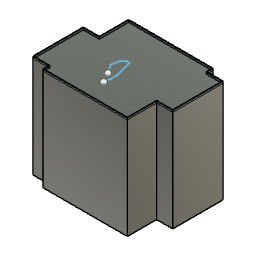
RSM_3d_model v1 (Autodesk Fusion 360 design; units mm, degrees)
Autodesk Fusion 360 part; units mm, degrees
sketch "Sketch1" plane through (0, 0, 0) normal (0, 0, 1) x (1, 0, 0)
sketch "Sketch2" plane through (0, 0, 0) normal (0, 0, 1) x (1, 0, 0)
  line L0 (106.508, 35.5843) -> (319.36, 35.5843)
  line L1 (106.508, 35.5843) -> (106.508, 50.8243)
  line L2 (106.508, 50.8243) -> (65.868, 50.8243)
  line L3 (65.868, 50.8243) -> (65.868, 177.8243)
  line L4 (65.868, 177.8243) -> (106.508, 177.8243)
  line L5 (106.508, 177.8243) -> (106.508, 251.4843)
  line L6 (106.508, 251.4843) -> (319.36, 251.4843)
  line L7 (319.36, 251.4843) -> (319.36, 236.2443)
  line L8 (319.36, 236.2443) -> (360, 236.2443)
  line L9 (360, 236.2443) -> (360, 109.2443)
  line L10 (360, 109.2443) -> (319.36, 109.2443)
  line L11 (319.36, 109.2443) -> (319.36, 35.5843)
  dimension "d2" = 212.852
  dimension "d3" = 15.24
  dimension "d4" = 40.64
  dimension "d5" = 127
  dimension "d6" = 40.64
  dimension "d7" = 73.66
  dimension "d8" = 212.852
  dimension "d9" = 15.24
  dimension "d10" = 40.64
  dimension "d11" = 73.66
  constraint horizontal L0
  constraint perpendicular L0 L1
  constraint perpendicular L1 L2
  constraint perpendicular L2 L3
  constraint perpendicular L3 L4
  constraint perpendicular L4 L5
  constraint perpendicular L5 L6
  constraint perpendicular L6 L7
  constraint perpendicular L7 L8
  constraint perpendicular L8 L9
  constraint perpendicular L9 L10
  constraint perpendicular L0 L11
  measures "d2" distance of L0.start L0.end
  measures "d3" distance of L0.start L1.end
  measures "d4" distance of L1.end L2.end
  measures "d5" distance of L2.end L3.end
  measures "d6" distance of L3.end L4.end
  measures "d7" distance of L4.end L5.end
  measures "d8" distance of L5.end L6.end
  measures "d9" distance of L6.end L7.end
  measures "d10" distance of L7.end L8.end
  measures "d11" distance of L0.end L10.end
extrude "Extrude1" add sketch "Sketch2" along normal blind 254
sketch "Sketch3" plane through (0, 0, 254) normal (0, 0, 1) x (-1, 0, 0)
  line L0 (-106.508, -35.5843) -> (-319.36, -35.5843)
  line L1 (-319.36, -35.5843) -> (-319.36, -109.2443)
  line L2 (-319.36, -109.2443) -> (-360, -109.2443)
  line L3 (-360, -109.2443) -> (-360, -236.2443)
  line L4 (-360, -236.2443) -> (-319.36, -236.2443)
  line L5 (-319.36, -236.2443) -> (-319.36, -251.4843)
  line L6 (-319.36, -251.4843) -> (-106.508, -251.4843)
  line L7 (-106.508, -251.4843) -> (-106.508, -177.8243)
  line L8 (-106.508, -177.8243) -> (-65.868, -177.8243)
  line L9 (-65.868, -177.8243) -> (-65.868, -50.8243)
  line L10 (-65.868, -50.8243) -> (-106.508, -50.8243)
  line L11 (-106.508, -50.8243) -> (-106.508, -35.5843)
  line L12 (-65.868, -177.8243) -> (-66.868, -177.8243)
  line L13 (-66.868, -177.8243) -> (-66.868, -50.8243)
  line L14 (-66.868, -50.8243) -> (-65.868, -50.8243)
  line L15 (-65.868, -50.8243) -> (-65.868, -177.8243)
  line L16 (-65.868, -177.8243) -> (-107.508, -177.8243)
  line L17 (-107.508, -177.8243) -> (-107.508, -176.8243)
  line L18 (-107.508, -176.8243) -> (-65.868, -176.8243)
  line L19 (-65.868, -176.8243) -> (-65.868, -177.8243)
  line L20 (-65.868, -50.8243) -> (-107.508, -50.8243)
  line L21 (-107.508, -50.8243) -> (-107.508, -51.8243)
  line L22 (-107.508, -51.8243) -> (-65.868, -51.8243)
  line L23 (-65.868, -51.8243) -> (-65.868, -50.8243)
  line L24 (-107.508, -51.8243) -> (-106.508, -51.8243)
  line L25 (-106.508, -51.8243) -> (-106.508, -35.5843)
  line L26 (-106.508, -35.5843) -> (-107.508, -35.5843)
  line L27 (-107.508, -35.5843) -> (-107.508, -51.8243)
  line L28 (-106.508, -35.5843) -> (-319.36, -35.5843)
  line L29 (-319.36, -35.5843) -> (-319.36, -36.5843)
  line L30 (-319.36, -36.5843) -> (-106.508, -36.5843)
  line L31 (-106.508, -36.5843) -> (-106.508, -35.5843)
  line L32 (-319.36, -35.5843) -> (-318.36, -35.5843)
  line L33 (-318.36, -35.5843) -> (-318.36, -110.2443)
  line L34 (-318.36, -110.2443) -> (-319.36, -110.2443)
  line L35 (-319.36, -110.2443) -> (-319.36, -35.5843)
  line L36 (-318.36, -110.2443) -> (-360, -110.2443)
  line L37 (-360, -110.2443) -> (-360, -109.2443)
  line L38 (-360, -109.2443) -> (-318.36, -109.2443)
  line L39 (-318.36, -109.2443) -> (-318.36, -110.2443)
  line L40 (-360, -236.2443) -> (-359, -236.2443)
  line L41 (-359, -236.2443) -> (-359, -109.2443)
  line L42 (-359, -109.2443) -> (-360, -109.2443)
  line L43 (-360, -109.2443) -> (-360, -236.2443)
  line L44 (-360, -236.2443) -> (-318.36, -236.2443)
  line L45 (-318.36, -236.2443) -> (-318.36, -235.2443)
  line L46 (-318.36, -235.2443) -> (-360, -235.2443)
  line L47 (-360, -235.2443) -> (-360, -236.2443)
  line L48 (-319.36, -251.4843) -> (-318.36, -251.4843)
  line L49 (-318.36, -251.4843) -> (-318.36, -235.2443)
  line L50 (-318.36, -235.2443) -> (-319.36, -235.2443)
  line L51 (-319.36, -235.2443) -> (-319.36, -251.4843)
  line L52 (-319.36, -251.4843) -> (-106.508, -251.4843)
  line L53 (-106.508, -251.4843) -> (-106.508, -250.4843)
  line L54 (-106.508, -250.4843) -> (-319.36, -250.4843)
  line L55 (-319.36, -250.4843) -> (-319.36, -251.4843)
  line L56 (-107.508, -176.8243) -> (-106.508, -176.8243)
  line L57 (-106.508, -176.8243) -> (-106.508, -251.4843)
  line L58 (-106.508, -251.4843) -> (-107.508, -251.4843)
  line L59 (-107.508, -251.4843) -> (-107.508, -176.8243)
  dimension "d14" = 1
  dimension "d15" = 1
  dimension "d16" = 1
  dimension "d17" = 1
  dimension "d18" = 1
  dimension "d19" = 1
  dimension "d20" = 1
  dimension "d21" = 1
  dimension "d22" = 1
  dimension "d23" = 1
  dimension "d24" = 1
  dimension "d25" = 1
  constraint horizontal L12
  constraint vertical L13
  constraint horizontal L14
  constraint vertical L15
  constraint coincident L10 L13.end
  constraint coincident L8.end L9.start
  constraint horizontal L16
  constraint vertical L17
  constraint horizontal L18
  constraint vertical L19
  constraint horizontal L20
  constraint vertical L21
  constraint horizontal L22
  constraint vertical L23
  constraint coincident L9.end L10.start
  constraint horizontal L24
  constraint vertical L25
  constraint horizontal L26
  constraint vertical L27
  constraint coincident L0.start L11.end
  constraint horizontal L28
  constraint vertical L29
  constraint horizontal L30
  constraint vertical L31
  constraint coincident L1 L29.end
  constraint horizontal L32
  constraint vertical L33
  constraint horizontal L34
  constraint vertical L35
  constraint horizontal L36
  constraint vertical L37
  constraint horizontal L38
  constraint vertical L39
  constraint coincident L2.end L3.start
  constraint horizontal L40
  constraint vertical L41
  constraint horizontal L42
  constraint vertical L43
  constraint coincident L2 L41.end
  constraint coincident L3.end L4.start
  constraint horizontal L44
  constraint vertical L45
  constraint horizontal L46
  constraint vertical L47
  constraint horizontal L48
  constraint vertical L49
  constraint horizontal L50
  constraint vertical L51
  constraint coincident L5.end L6.start
  constraint horizontal L52
  constraint vertical L53
  constraint horizontal L54
  constraint vertical L55
  constraint coincident L7 L53.end
  constraint horizontal L56
  constraint vertical L57
  constraint horizontal L58
  constraint vertical L59
  constraint coincident L6.end L7.start
  measures "d14" distance of L8.end L12.end
  measures "d15" distance of L8.end L18.end
  measures "d16" distance of L53.end L6.end
  measures "d17" distance of L6.end L58.end
  measures "d18" distance of L5.end L48.end
  measures "d19" distance of L44.end L45.end
  measures "d20" distance of L3.end L40.end
  measures "d21" distance of L36.end L2.end
  measures "d22" distance of L33.end L34.end
  measures "d23" distance of L20.end L21.end
  measures "d24" distance of L21.end L24.end
  measures "d25" distance of L0.start L30.end
extrude "Extrude2" add sketch "Sketch3" along normal blind 5 contours L0 L11 L25 L26 L27 L28 L30 L31 | L0 L27 L28 L30 L33 | L11 L20 L25 L27 L30 | L0 L1 L28 L29 L30 L32 L33 L35 | L20 L21 L22 L24 L25 L27 | L10 L13 L20 L22 L25 | L1 L30 L33 L35 L38 | L9 L10 L13 L14 L15 L20 L22 L23 | L33 L34 L35 L36 L38 L39 | L9 L13 L15 L18 L22 | L2 L35 L36 L38 L41 | L8 L9 L12 L13 L15 L16 L18 L19 | L8 L13 L16 L18 L57 | L2 L3 L36 L37 L38 L41 L42 L43 | L16 L17 L18 L56 L57 L59 | L3 L36 L41 L43 L46 | L7 L16 L54 L57 L59 | L4 L41 L44 L46 L51 | L3 L4 L40 L41 L43 L44 L46 L47 | L6 L7 L52 L53 L54 L57 L58 L59 | L44 L45 L46 L49 L50 L51 | L6 L49 L52 L54 L59 | L5 L44 L49 L51 L54 | L5 L6 L48 L49 L51 L52 L54 L55
sketch "Sketch4" plane through (0, 0, 254) normal (0, 0, 1) x (-1, 0, 0)
  line L0 (-107.508, -176.8243) -> (-66.868, -176.8243)
  line L1 (-66.868, -176.8243) -> (-66.868, -51.8243)
  line L2 (-66.868, -51.8243) -> (-107.508, -51.8243)
  line L3 (-107.508, -51.8243) -> (-107.508, -36.5843)
  line L4 (-107.508, -36.5843) -> (-318.36, -36.5843)
  line L5 (-318.36, -36.5843) -> (-318.36, -110.2443)
  line L6 (-318.36, -110.2443) -> (-359, -110.2443)
  line L7 (-359, -110.2443) -> (-359, -235.2443)
  line L8 (-359, -235.2443) -> (-318.36, -235.2443)
  line L9 (-318.36, -235.2443) -> (-318.36, -250.4843)
  line L10 (-318.36, -250.4843) -> (-107.508, -250.4843)
  line L11 (-107.508, -250.4843) -> (-107.508, -176.8243)
  line L12 (-192.7092, -113.2958) -> (-177.8821, -135.8603)
  line L13 (-177.8821, -135.8603) -> (-181.5924, -155.5132)
  line L14 (-181.5924, -155.5132) -> (-189.7272, -162.9176)
  line L15 (-189.7272, -162.9176) -> (-197.3239, -162.6933)
  line L16 (-197.3239, -162.6933) -> (-208.6768, -121.2191)
  line L17 (-208.6768, -121.2191) -> (-209.0766, -103.7236)
  line L18 (-209.0766, -103.7236) -> (-206.2382, -88.6892)
  dimension "d40" = 27
  dimension "d42" = 11
  dimension "d44" = 43
  dimension "d46" = 17.5
  dimension "d47" = 7.6
  dimension "d48" = 107
  dimension "d49" = 166
  dimension "d50" = 20
  dimension "d51" = 136
  dimension "d52" = 143
  dimension "d54" = 15.3
  dimension "d55" = 168
  constraint parallel L13 L18
  measures "d40" distance of L12.start L12.end
  measures "d42" distance of L13.end L14.end
  measures "d44" distance of L15.end L16.end
  measures "d46" distance of L16.end L17.end
  measures "d47" distance of L14.end L15.end
  measures "d48" angle of L15 L16
  measures "d49" angle of L16 L17
  measures "d50" distance of L12.end L13.end
  measures "d51" angle of L12 L13
  measures "d52" angle of L13 L14
  measures "d54" distance of L17.end L18.end
  measures "d55" angle of L17 L18
